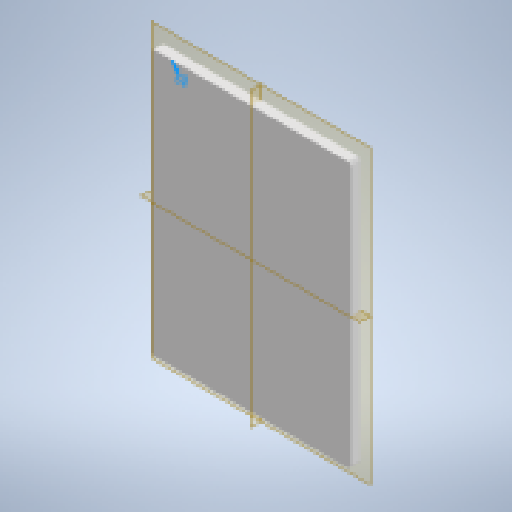
# Autodesk Inventor part: Mesa_ergonomica
Saved by Autodesk Inventor 2025.2 (Build 292293000, 293)
## iProperties
Created: 2025-04-02
Part Number: Mesa_ergonomica
Material: Generic
Document SubType Name: Modeling
Designer: ishad
Density: 1 g/cm^3
Appearance: Default
Author: ishad
Autodesk Inventor part; units mm, degrees
sketch "Sketch1" plane through (0, 0, 0) normal (0, 0, 1) x (1, 0, 0)
  line L0 (300, -400) -> (-300, -400)
  line L1 (-300, -400) -> (-300, 400)
  line L2 (-300, 400) -> (300, 400)
  line L3 (300, 400) -> (300, -400)
  line L4 (300, -400) -> (-300, 400) construction
  line L5 (-300, -400) -> (300, 400) construction
  point P0 (0, 0)
  dimension "d1" = 600
  dimension "d2" = 800
  constraints: 12 end point, 2 midpoint, 2 parallel, 1 horizontal, 1 perpendicular
  measures "d1" distance of L1.end L2.end
  measures "d2" distance between parallel lines of L0 L2
extrude "Extrusion1" add sketch "Sketch1" along normal mid plane 30
fillet "Fillet1" radius 10 1 edges at (300, 400, 0)
fillet "Fillet2" radius 10 1 edges at (300, -400, 0)
fillet "Fillet3" radius 10 2 edges at (-300, -400, 0) (-300, 400, 0)
sketch "Sketch6" plane through (0, 0, 0) normal (0, 0, 1) x (1, 0, 0)
  line L0 (-300, -390) -> (-300, 390) projected
  line L1 (-290, 400) -> (290, 400) projected
  circle A0 centre (-250, 341) radius 29.946
  point P0 (0, 0)
  dimension "d29" = 50
  dimension "d30" = 59
  constraints: 1 centre point
  measures "d29" distance from line of L0 A0.centre
  measures "d30" distance from line of L1 A0.centre
sketch "Sketch7" plane through (0, 0, 0) normal (0, 0, 1) x (1, 0, 0)
  point P0 (0, 0)
extrude "Extrusion3" cut sketch "Sketch6" against normal blind 30
body "Solid1"
